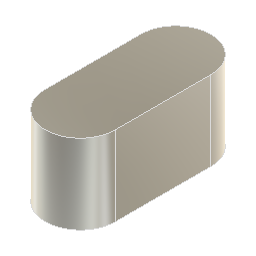
Паз для фиксации(Требуется 2) (Autodesk Fusion 360 design; units mm, degrees)
Autodesk Fusion 360 part; units mm, degrees
sketch "Sketch1" plane through (0, 0, 0) normal (0, 0, 1) x (1, 0, 0)
  line L0 (2.2, -3) -> (2.2, 3)
  arc A0 (2.2, 3) -> (-2.2, 3) centre (0, 3) ccw
  line L1 (-2.2, 3) -> (-2.2, -3)
  arc A1 (-2.2, -3) -> (2.2, -3) centre (0, -3) ccw
extrude "Extrude1" add sketch "Sketch1" along normal blind 5
